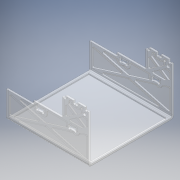
# Autodesk Inventor part: バッテリーボックス底板
Saved by Autodesk Inventor 2016 (Build 200138000, 138)
## iProperties
Created: 2019-03-23
Part Number: バッテリーボックス底板
Material: ポリカーボネート、クリア
Document SubType Name: Modeling
Designer: mozar
Density: 1.2 g/cm^3
Appearance: ポリカーボネート - クリア
Author: mozar
Autodesk Inventor part; units mm, degrees
note: some values were not read from the file. Chosen so that the rebuilt part matches the saved one: bend side of "曲げパーツ2".
(part 1 of 2)
ref_plane "YZ Plane" through (0, 0, 0) normal (1, 0, 0) x (0, 1, 0)
ref_plane "XZ Plane" through (0, 0, 0) normal (0, 1, 0) x (-1, 0, 0)
ref_plane "XY Plane" through (0, 0, 0) normal (0, 0, 1) x (1, 0, 0)
sketch "スケッチ1" plane through (0, 0, 0) normal (0, 0, 1) x (1, 0, 0)
  circle A0 centre (140, 30) radius 1.5
  circle A1 centre (140, -164.2) radius 1.5
  arc A2 (140.8182, -159.775) -> (142, -158.7917) centre (141, -158.7917) ccw
  line L0 (142, -158.7917) -> (142, -151.9032)
  arc A3 (142, -151.9032) -> (140.4377, -151.0763) centre (141, -151.9032) ccw
  line L1 (140.4377, -151.0763) -> (133.3836, -155.8731)
  arc A4 (133.3836, -155.8731) -> (133.3836, -157.5269) centre (133.9459, -156.7) ccw
  line L2 (133.3836, -157.5269) -> (137.0951, -160.0507)
  arc A5 (137.0951, -160.0507) -> (138.0834, -160.1286) centre (137.6574, -159.2238) ccw
  arc A6 (140.8182, -159.775) -> (138.0834, -160.1286) centre (140, -164.2) ccw
  arc A7 (136.2251, -169.2) -> (136.9114, -167.4727) centre (136.2251, -168.2) ccw
  arc A8 (136.7273, -167.2886) -> (136.9114, -167.4727) centre (140, -164.2) ccw
  arc A9 (136.7273, -167.2886) -> (135, -167.9749) centre (136, -167.9749) ccw
  line L3 (135, -167.9749) -> (135, -168.2)
  arc A10 (135, -168.2) -> (136, -169.2) centre (136, -168.2) ccw
  line L4 (136, -169.2) -> (136.2251, -169.2)
  arc A11 (136.9114, 33.2727) -> (136.2251, 35) centre (136.2251, 34) ccw
  line L5 (136.2251, 35) -> (136, 35)
  arc A12 (136, 35) -> (135, 34) centre (136, 34) ccw
  line L6 (135, 34) -> (135, 33.7749)
  arc A13 (135, 33.7749) -> (136.7273, 33.0886) centre (136, 33.7749) ccw
  arc A14 (136.9114, 33.2727) -> (136.7273, 33.0886) centre (140, 30) ccw
  arc A15 (140.4377, 16.8763) -> (142, 17.7032) centre (141, 17.7032) ccw
  line L7 (142, 17.7032) -> (142, 24.5917)
  arc A16 (142, 24.5917) -> (140.8182, 25.575) centre (141, 24.5917) ccw
  arc A17 (138.0834, 25.9286) -> (140.8182, 25.575) centre (140, 30) ccw
  arc A18 (138.0834, 25.9286) -> (137.0951, 25.8507) centre (137.6574, 25.0238) ccw
  line L8 (137.0951, 25.8507) -> (133.3836, 23.3269)
  arc A19 (133.3836, 23.3269) -> (133.3836, 21.6731) centre (133.9459, 22.5) ccw
  line L9 (133.3836, 21.6731) -> (140.4377, 16.8763)
  arc A20 (130.0623, 20.3037) -> (128.9377, 20.3037) centre (129.5, 19.4768) ccw
  line L10 (128.9377, 20.3037) -> (122.3542, 15.8269)
  arc A21 (122.3542, 15.8269) -> (122.9165, 14) centre (122.9165, 15) ccw
  line L11 (122.9165, 14) -> (136.0835, 14)
  arc A22 (136.0835, 14) -> (136.6458, 15.8269) centre (136.0835, 15) ccw
  line L12 (136.6458, 15.8269) -> (130.0623, 20.3037)
  arc A23 (121, 32) -> (120.7896, 30.237) centre (121.3519, 31.064) ccw
  line L13 (120.7896, 30.237) -> (128.9377, 24.6963)
  arc A24 (128.9377, 24.6963) -> (130.0623, 24.6963) centre (129.5, 25.5232) ccw
  line L14 (130.0623, 24.6963) -> (135.1564, 28.1603)
  arc A25 (135.1564, 28.1603) -> (135.577, 29.1713) centre (134.5941, 28.9872) ccw
  arc A26 (135.575, 30.8182) -> (135.577, 29.1713) centre (140, 30) ccw
  arc A27 (135.575, 30.8182) -> (134.5917, 32) centre (134.5917, 31) ccw
  line L15 (134.5917, 32) -> (134, 32)
  arc A28 (134, 32) -> (133.4, 31.8) centre (134, 31) ccw
  arc A29 (129.8, 31.1842) -> (133.4, 31.8) centre (131, 35) ccw
  arc A30 (129.8, 31.1842) -> (129.2, 31.1842) centre (129.5, 30.2303) ccw
  arc A31 (125.6, 31.8) -> (129.2, 31.1842) centre (128, 35) ccw
  arc A32 (125.6, 31.8) -> (125, 32) centre (125, 31) ccw
  line L16 (125, 32) -> (124, 32)
  line L17 (124, 32) -> (124, 34)
  arc A33 (124, 34) -> (123, 35) centre (123, 34) ccw
  line L18 (123, 35) -> (122, 35)
  arc A34 (122, 35) -> (121, 34) centre (122, 34) ccw
  line L19 (121, 34) -> (121, 32)
  arc A35 (117, 17.7032) -> (118.5623, 16.8763) centre (118, 17.7032) ccw
  line L20 (118.5623, 16.8763) -> (125.6164, 21.6731)
  arc A36 (125.6164, 21.6731) -> (125.6164, 23.3269) centre (125.0541, 22.5) ccw
  line L21 (125.6164, 23.3269) -> (118.5623, 28.1237)
  arc A37 (118.5623, 28.1237) -> (117, 27.2968) centre (118, 27.2968) ccw
  line L22 (117, 27.2968) -> (117, 17.7032)
  arc A38 (125, 4) -> (124.4, 3.8) centre (125, 3) ccw
  arc A39 (121.6491, 3.0154) -> (124.4, 3.8) centre (122, 7) ccw
  arc A40 (121.6491, 3.0154) -> (121.2641, 2.9741) centre (121.5614, 2.0193) ccw
  line L23 (121.2641, 2.9741) -> (101.9364, -3.0425)
  arc A41 (101.9364, -3.0425) -> (101.9774, -4.9639) centre (102.2336, -3.9973) ccw
  line L24 (101.9774, -4.9639) -> (140.7437, -15.2421)
  arc A42 (140.7437, -15.2421) -> (142, -14.2755) centre (141, -14.2755) ccw
  line L25 (142, -14.2755) -> (142, 8.0704)
  arc A43 (142, 8.0704) -> (140.7028, 9.0252) centre (141, 8.0704) ccw
  line L26 (140.7028, 9.0252) -> (133.5686, 6.8044)
  arc A44 (133.5686, 6.8044) -> (132.8927, 6.0797) centre (133.8659, 5.8496) ccw
  arc A45 (126.6, 3.8) -> (132.8927, 6.0797) centre (129, 7) ccw
  arc A46 (126.6, 3.8) -> (126, 4) centre (126, 3) ccw
  line L27 (126, 4) -> (125, 4)
  arc A47 (80.0808, 6.2) -> (79.101, 7) centre (79.101, 6) ccw
  line L28 (79.101, 7) -> (64.5268, 7)
  arc A48 (64.5268, 7) -> (64.2705, 5.0334) centre (64.5268, 6) ccw
  line L29 (64.2705, 5.0334) -> (92.8926, -2.5553)
  arc A49 (92.8926, -2.5553) -> (93.4461, -2.5435) centre (93.1489, -1.5887) ccw
  line L30 (93.4461, -2.5435) -> (117.4252, 4.9211)
  arc A50 (117.4252, 4.9211) -> (118.1024, 6.1007) centre (117.128, 5.8759) ccw
  arc A51 (118, 7) -> (118.1024, 6.1007) centre (122, 7) ccw
  line L31 (118, 7) -> (118, 10)
  arc A52 (118, 10) -> (117, 11) centre (117, 10) ccw
  line L32 (117, 11) -> (96, 11)
  arc A53 (96, 11) -> (95, 10) centre (96, 10) ccw
  line L33 (95, 10) -> (95, 7)
  arc A54 (88.6, 3.8) -> (95, 7) centre (91, 7) ccw
  arc A55 (88.6, 3.8) -> (88, 4) centre (88, 3) ccw
  line L34 (88, 4) -> (87, 4)
  arc A56 (87, 4) -> (86.4, 3.8) centre (87, 3) ccw
  arc A57 (80.0808, 6.2) -> (86.4, 3.8) centre (84, 7) ccw
  arc A58 (52.2563, 5.1151) -> (51, 4.1485) centre (52, 4.1485) ccw
  line L35 (51, 4.1485) -> (51, -14.398)
  arc A59 (51, -14.398) -> (52.2972, -15.3528) centre (52, -14.398) ccw
  line L36 (52.2972, -15.3528) -> (84.4723, -5.337)
  arc A60 (84.4723, -5.337) -> (84.4313, -3.4155) centre (84.1751, -4.3821) ccw
  line L37 (84.4313, -3.4155) -> (52.2563, 5.1151)
  arc A61 (127.9942, -17) -> (128.2505, -15.0334) centre (127.9942, -16) ccw
  line L38 (128.2505, -15.0334) -> (93.5161, -5.8242)
  arc A62 (93.5161, -5.8242) -> (92.9626, -5.836) centre (93.2598, -6.7908) ccw
  line L39 (92.9626, -5.836) -> (63.3788, -15.0452)
  arc A63 (63.3788, -15.0452) -> (63.676, -17) centre (63.676, -16) ccw
  line L40 (63.676, -17) -> (127.9942, -17)
  arc A64 (128.2505, -119.1666) -> (127.9942, -117.2) centre (127.9942, -118.2) ccw
  line L41 (127.9942, -117.2) -> (63.1515, -117.2)
  arc A65 (63.1515, -117.2) -> (62.8561, -119.1554) centre (63.1515, -118.2) ccw
  line L42 (62.8561, -119.1554) -> (92.7876, -128.4114)
  arc A66 (92.7876, -128.4114) -> (93.3393, -128.4227) centre (93.0831, -127.4561) ccw
  line L43 (93.3393, -128.4227) -> (128.2505, -119.1666)
  arc A67 (51, -138.3485) -> (52.2563, -139.3151) centre (52, -138.3485) ccw
  line L44 (52.2563, -139.3151) -> (84.2275, -130.8385)
  arc A68 (84.2275, -130.8385) -> (84.2666, -128.9165) centre (83.9712, -129.8719) ccw
  line L45 (84.2666, -128.9165) -> (52.2954, -119.0297)
  arc A69 (52.2954, -119.0297) -> (51, -119.9851) centre (52, -119.9851) ccw
  line L46 (51, -119.9851) -> (51, -138.3485)
  arc A70 (123, -169.2) -> (124, -168.2) centre (123, -168.2) ccw
  line L47 (124, -168.2) -> (124, -166.2)
  line L48 (124, -166.2) -> (125, -166.2)
  arc A71 (125, -166.2) -> (125.6, -166) centre (125, -165.2) ccw
  arc A72 (129.2, -165.3842) -> (125.6, -166) centre (128, -169.2) ccw
  arc A73 (129.2, -165.3842) -> (129.8, -165.3842) centre (129.5, -164.4303) ccw
  arc A74 (133.4, -166) -> (129.8, -165.3842) centre (131, -169.2) ccw
  arc A75 (133.4, -166) -> (134, -166.2) centre (134, -165.2) ccw
  line L49 (134, -166.2) -> (134.5917, -166.2)
  arc A76 (134.5917, -166.2) -> (135.575, -165.0182) centre (134.5917, -165.2) ccw
  arc A77 (135.577, -163.3713) -> (135.575, -165.0182) centre (140, -164.2) ccw
  arc A78 (135.577, -163.3713) -> (135.1564, -162.3603) centre (134.5941, -163.1872) ccw
  line L50 (135.1564, -162.3603) -> (130.0623, -158.8963)
  arc A79 (130.0623, -158.8963) -> (128.9377, -158.8963) centre (129.5, -159.7232) ccw
  line L51 (128.9377, -158.8963) -> (120.7896, -164.437)
  arc A80 (120.7896, -164.437) -> (121, -166.2) centre (121.3519, -165.264) ccw
  line L52 (121, -166.2) -> (121, -168.2)
  arc A81 (121, -168.2) -> (122, -169.2) centre (122, -168.2) ccw
  line L53 (122, -169.2) -> (123, -169.2)
  arc A82 (125.6164, -157.5269) -> (125.6164, -155.8731) centre (125.0541, -156.7) ccw
  line L54 (125.6164, -155.8731) -> (118.5623, -151.0763)
  arc A83 (118.5623, -151.0763) -> (117, -151.9032) centre (118, -151.9032) ccw
  line L55 (117, -151.9032) -> (117, -161.4968)
  arc A84 (117, -161.4968) -> (118.5623, -162.3237) centre (118, -161.4968) ccw
  line L56 (118.5623, -162.3237) -> (125.6164, -157.5269)
  arc A85 (122.9165, -148.2) -> (122.3542, -150.0269) centre (122.9165, -149.2) ccw
  line L57 (122.3542, -150.0269) -> (128.9377, -154.5037)
  arc A86 (128.9377, -154.5037) -> (130.0623, -154.5037) centre (129.5, -153.6768) ccw
  line L58 (130.0623, -154.5037) -> (136.6458, -150.0269)
  arc A87 (136.6458, -150.0269) -> (136.0835, -148.2) centre (136.0835, -149.2) ccw
  line L59 (136.0835, -148.2) -> (122.9165, -148.2)
  arc A88 (121.1595, -137.1852) -> (121.5639, -137.2238) centre (121.4549, -136.2298) ccw
  arc A89 (124.4, -138) -> (121.5639, -137.2238) centre (122, -141.2) ccw
  arc A90 (124.4, -138) -> (125, -138.2) centre (125, -137.2) ccw
  line L60 (125, -138.2) -> (126, -138.2)
  arc A91 (126, -138.2) -> (126.6, -138) centre (126, -137.2) ccw
  arc A92 (132.8964, -140.2954) -> (126.6, -138) centre (129, -141.2) ccw
  arc A93 (132.8964, -140.2954) -> (133.575, -141.0246) centre (133.8705, -140.0692) ccw
  line L61 (133.575, -141.0246) -> (140.7046, -143.2293)
  arc A94 (140.7046, -143.2293) -> (142, -142.2739) centre (141, -142.2739) ccw
  line L62 (142, -142.2739) -> (142, -119.9245)
  arc A95 (142, -119.9245) -> (140.7437, -118.9579) centre (141, -119.9245) ccw
  line L63 (140.7437, -118.9579) -> (101.8327, -129.2745)
  arc A96 (101.8327, -129.2745) -> (101.7935, -131.1964) centre (102.089, -130.2411) ccw
  line L64 (101.7935, -131.1964) -> (121.1595, -137.1852)
  arc A97 (117, -145.2) -> (118, -144.2) centre (117, -144.2) ccw
  line L65 (118, -144.2) -> (118, -141.2)
  arc A98 (118.094, -140.3377) -> (118, -141.2) centre (122, -141.2) ccw
  arc A99 (118.094, -140.3377) -> (117.413, -139.1668) centre (117.1176, -140.1221) ccw
  line L66 (117.413, -139.1668) -> (93.2725, -131.7015)
  arc A100 (93.2725, -131.7015) -> (92.7208, -131.6903) centre (92.9771, -132.6569) ccw
  line L67 (92.7208, -131.6903) -> (64.2705, -139.2334)
  arc A101 (64.2705, -139.2334) -> (64.5268, -141.2) centre (64.5268, -140.2) ccw
  line L68 (64.5268, -141.2) -> (79.101, -141.2)
  arc A102 (79.101, -141.2) -> (80.0808, -140.4) centre (79.101, -140.2) ccw
  arc A103 (86.4, -138) -> (80.0808, -140.4) centre (84, -141.2) ccw
  arc A104 (86.4, -138) -> (87, -138.2) centre (87, -137.2) ccw
  line L69 (87, -138.2) -> (88, -138.2)
  arc A105 (88, -138.2) -> (88.6, -138) centre (88, -137.2) ccw
  arc A106 (95, -141.2) -> (88.6, -138) centre (91, -141.2) ccw
  line L70 (95, -141.2) -> (95, -144.2)
  arc A107 (95, -144.2) -> (96, -145.2) centre (96, -144.2) ccw
  line L71 (96, -145.2) -> (117, -145.2)
  arc A108 (128, -144.2) -> (130, -144.2) centre (129, -144.2) ccw
  line L72 (130, -144.2) -> (130, -141.2)
  arc A109 (130, -141.2) -> (128, -141.2) centre (129, -141.2) ccw
  line L73 (128, -141.2) -> (123, -141.2)
  arc A110 (123, -141.2) -> (121, -141.2) centre (122, -141.2) ccw
  line L74 (121, -141.2) -> (121, -144.2)
  arc A111 (121, -144.2) -> (123, -144.2) centre (122, -144.2) ccw
  line L75 (123, -144.2) -> (128, -144.2)
  arc A112 (90, 7) -> (92, 7) centre (91, 7) ccw
  line L76 (92, 7) -> (92, 10)
  arc A113 (92, 10) -> (90, 10) centre (91, 10) ccw
  line L77 (90, 10) -> (85, 10)
  arc A114 (85, 10) -> (83, 10) centre (84, 10) ccw
  line L78 (83, 10) -> (83, 7)
  arc A115 (83, 7) -> (85, 7) centre (84, 7) ccw
  line L79 (85, 7) -> (90, 7)
  arc A116 (121, 7) -> (123, 7) centre (122, 7) ccw
  line L80 (123, 7) -> (128, 7)
  arc A117 (128, 7) -> (130, 7) centre (129, 7) ccw
  line L81 (130, 7) -> (130, 10)
  arc A118 (130, 10) -> (128, 10) centre (129, 10) ccw
  line L82 (128, 10) -> (123, 10)
  arc A119 (123, 10) -> (121, 10) centre (122, 10) ccw
  line L83 (121, 10) -> (121, 7)
  arc A120 (83, -144.2) -> (85, -144.2) centre (84, -144.2) ccw
  line L84 (85, -144.2) -> (90, -144.2)
  arc A121 (90, -144.2) -> (92, -144.2) centre (91, -144.2) ccw
  line L85 (92, -144.2) -> (92, -141.2)
  arc A122 (92, -141.2) -> (90, -141.2) centre (91, -141.2) ccw
  line L86 (90, -141.2) -> (85, -141.2)
  arc A123 (85, -141.2) -> (83, -141.2) centre (84, -141.2) ccw
  line L87 (83, -141.2) -> (83, -144.2)
  arc A124 (24.5071, -36.0492) -> (23.2695, -35.6053) centre (23.6339, -36.5366) ccw
  line L88 (23.2695, -35.6053) -> (2.9387, -43.5608)
  arc A125 (2.9387, -43.5608) -> (3.0119, -45.4487) centre (3.3031, -44.4921) ccw
  line L89 (3.0119, -45.4487) -> (22.9517, -51.5174)
  arc A126 (22.9517, -51.5174) -> (24.1943, -50.8686) centre (23.2428, -50.5607) ccw
  arc A127 (25.7746, -48.7762) -> (24.1943, -50.8686) centre (28, -52.1) ccw
  line L90 (25.7746, -48.7762) -> (26, -48.1)
  line L91 (26, -48.1) -> (32, -48.1)
  arc A128 (32, -48.1) -> (33, -47.1) centre (32, -47.1) ccw
  line L92 (33, -47.1) -> (33, -39.1)
  arc A129 (33, -39.1) -> (32, -38.1) centre (32, -39.1) ccw
  line L93 (32, -38.1) -> (26, -38.1)
  line L94 (26, -38.1) -> (25.8761, -37.7283)
  arc A130 (25.8761, -37.7283) -> (25.5419, -37.2556) centre (24.9274, -38.0445) ccw
  arc A131 (24.5071, -36.0492) -> (25.5419, -37.2556) centre (28, -34.1) ccw
  arc A132 (-24.4188, -35.8819) -> (-23.8147, -37.2841) centre (-23.5236, -36.3274) ccw
  line L95 (-23.8147, -37.2841) -> (-4.7062, -43.0997)
  arc A133 (-4.7062, -43.0997) -> (-4.0507, -43.0743) centre (-4.4151, -42.1431) ccw
  line L96 (-4.0507, -43.0743) -> (12.6705, -36.5312)
  arc A134 (12.6705, -36.5312) -> (12.3061, -34.6) centre (12.3061, -35.6) ccw
  line L97 (12.3061, -34.6) -> (-23.2303, -34.6)
  arc A135 (-23.2303, -34.6) -> (-24.1842, -35.3) centre (-23.2303, -35.6) ccw
  arc A136 (-24.4188, -35.8819) -> (-24.1842, -35.3) centre (-28, -34.1) ccw
  arc A137 (-3.9188, -46.4753) -> (-4.5743, -46.5007) centre (-4.2099, -47.4319) ccw
  line L98 (-4.5743, -46.5007) -> (-12.6705, -49.6688)
  arc A138 (-12.6705, -49.6688) -> (-12.3061, -51.6) centre (-12.3061, -50.6) ccw
  line L99 (-12.3061, -51.6) -> (6.1994, -51.6)
  arc A139 (6.1994, -51.6) -> (6.4906, -49.6433) centre (6.1994, -50.6) ccw
  line L100 (6.4906, -49.6433) -> (-3.9188, -46.4753)
  arc A140 (-24.5071, -50.1508) -> (-23.2695, -50.5947) centre (-23.6339, -49.6634) ccw
  line L101 (-23.2695, -50.5947) -> (-11.5637, -46.0142)
  arc A141 (-11.5637, -46.0142) -> (-11.6369, -44.1263) centre (-11.9281, -45.0829) ccw
  line L102 (-11.6369, -44.1263) -> (-28.7088, -38.9305)
  arc A142 (-28.7088, -38.9305) -> (-30, -39.8871) centre (-29, -39.8871) ccw
  line L103 (-30, -39.8871) -> (-30, -40.1)
  line L104 (-30, -40.1) -> (-32, -40.1)
  arc A143 (-32, -40.1) -> (-33, -41.1) centre (-32, -41.1) ccw
  line L105 (-33, -41.1) -> (-33, -47.1)
  arc A144 (-33, -47.1) -> (-32, -48.1) centre (-32, -47.1) ccw
  line L106 (-32, -48.1) -> (-26, -48.1)
  line L107 (-26, -48.1) -> (-25.8761, -48.4717)
  arc A145 (-25.8761, -48.4717) -> (-25.5419, -48.9444) centre (-24.9274, -48.1555) ccw
  arc A146 (-24.5071, -50.1508) -> (-25.5419, -48.9444) centre (-28, -52.1) ccw
  arc A147 (-44.8158, -35.3) -> (-45.7697, -34.6) centre (-45.7697, -35.6) ccw
  line L108 (-45.7697, -34.6) -> (-49, -34.6)
  line L109 (-49, -34.6) -> (-49, -50.6)
  arc A148 (-49, -50.6) -> (-48, -51.6) centre (-48, -50.6) ccw
  line L110 (-48, -51.6) -> (-45.7697, -51.6)
  arc A149 (-45.7697, -51.6) -> (-44.8158, -50.9) centre (-45.7697, -50.6) ccw
  arc A150 (-43.4581, -48.9444) -> (-44.8158, -50.9) centre (-41, -52.1) ccw
  arc A151 (-43.4581, -48.9444) -> (-43.1239, -48.4717) centre (-44.0726, -48.1555) ccw
  line L111 (-43.1239, -48.4717) -> (-43, -48.1)
  line L112 (-43, -48.1) -> (-37, -48.1)
  arc A152 (-37, -48.1) -> (-36, -47.1) centre (-37, -47.1) ccw
  line L113 (-36, -47.1) -> (-36, -41.1)
  arc A153 (-36, -41.1) -> (-37, -40.1) centre (-37, -41.1) ccw
  line L114 (-37, -40.1) -> (-39, -40.1)
  line L115 (-39, -40.1) -> (-39, -38.999)
  arc A154 (-39, -38.999) -> (-40.2, -38.0192) centre (-40, -38.999) ccw
  arc A155 (-44.8158, -35.3) -> (-40.2, -38.0192) centre (-41, -34.1) ccw
  arc A156 (-33.9671, -24.899) -> (-35.1671, -23.9192) centre (-34.9671, -24.899) ccw
  arc A157 (-38.3671, -23.2) -> (-35.1671, -23.9192) centre (-35.9671, -20) ccw
  arc A158 (-38.3671, -23.2) -> (-38.9671, -23) centre (-38.9671, -24) ccw
  line L116 (-38.9671, -23) -> (-48, -23)
  arc A159 (-48, -23) -> (-49, -24) centre (-48, -24) ccw
  line L117 (-49, -24) -> (-49, -29.6)
  arc A160 (-49, -29.6) -> (-48, -30.6) centre (-48, -29.6) ccw
  line L118 (-48, -30.6) -> (-45.7697, -30.6)
  arc A161 (-45.7697, -30.6) -> (-44.8158, -29.9) centre (-45.7697, -29.6) ccw
  arc A162 (-43.4581, -27.9444) -> (-44.8158, -29.9) centre (-41, -31.1) ccw
  arc A163 (-43.4581, -27.9444) -> (-43.1239, -27.4717) centre (-44.0726, -27.1555) ccw
  line L119 (-43.1239, -27.4717) -> (-43, -27.1)
  line L120 (-43, -27.1) -> (-34.962, -27.1)
  arc A164 (-34.962, -27.1) -> (-33.9671, -26) centre (-34.962, -26.1) ccw
  line L121 (-33.9671, -26) -> (-33.9671, -24.899)
  arc A165 (14.3908, -24.607) -> (15.2527, -25.1) centre (15.2527, -24.1) ccw
  line L122 (15.2527, -25.1) -> (44.4281, -25.1)
  arc A166 (44.4281, -25.1) -> (45.29, -24.607) centre (44.4281, -24.1) ccw
  line L123 (45.29, -24.607) -> (47.8619, -20.2347)
  line L124 (48, -19.7277) -> (48, 10)
  line L125 (48, 10) -> (79, 10)
  arc A167 (79, 10) -> (80, 11) centre (79, 11) ccw
  line L126 (80, 11) -> (80, 14)
  line L127 (80, 14) -> (113, 14)
  arc A168 (113, 14) -> (114, 15) centre (113, 15) ccw
  line L128 (114, 15) -> (114, 35)
  line L129 (114, 35) -> (116, 35)
  arc A169 (116, 35) -> (118, 35) centre (117, 35) ccw
  line L130 (118, 35) -> (118, 38)
  line L131 (118, 38) -> (127, 38)
  line L132 (127, 38) -> (127, 35)
  arc A170 (127, 35) -> (129, 35) centre (128, 35) ccw
  line L133 (129, 35) -> (130, 35)
  arc A171 (130, 35) -> (132, 35) centre (131, 35) ccw
  line L134 (132, 35) -> (132, 38)
  line L135 (132, 38) -> (141, 38)
  line L136 (141, 38) -> (141, 35)
  arc A172 (141, 35) -> (143, 35) centre (142, 35) ccw
  line L137 (143, 35) -> (145, 35)
  line L138 (145, 35) -> (145, -169.2)
  line L139 (145, -169.2) -> (143, -169.2)
  arc A173 (143, -169.2) -> (141, -169.2) centre (142, -169.2) ccw
  line L140 (141, -169.2) -> (141, -172.2)
  line L141 (141, -172.2) -> (132, -172.2)
  line L142 (132, -172.2) -> (132, -169.2)
  arc A174 (132, -169.2) -> (130, -169.2) centre (131, -169.2) ccw
  line L143 (130, -169.2) -> (129, -169.2)
  arc A175 (129, -169.2) -> (127, -169.2) centre (128, -169.2) ccw
  line L144 (127, -169.2) -> (127, -172.2)
  line L145 (127, -172.2) -> (118, -172.2)
  line L146 (118, -172.2) -> (118, -169.2)
  arc A176 (118, -169.2) -> (116, -169.2) centre (117, -169.2) ccw
  line L147 (116, -169.2) -> (114, -169.2)
  line L148 (114, -169.2) -> (114, -149.2)
  arc A177 (114, -149.2) -> (113, -148.2) centre (113, -149.2) ccw
  line L149 (113, -148.2) -> (80, -148.2)
  line L150 (80, -148.2) -> (80, -145.2)
  arc A178 (80, -145.2) -> (79, -144.2) centre (79, -145.2) ccw
  line L151 (79, -144.2) -> (48, -144.2)
  line L152 (48, -144.2) -> (48, -114.4723)
  line L153 (47.8619, -113.9653) -> (45.29, -109.593)
  arc A179 (45.29, -109.593) -> (44.4281, -109.1) centre (44.4281, -110.1) ccw
  line L154 (44.4281, -109.1) -> (15.2527, -109.1)
  arc A180 (15.2527, -109.1) -> (14.3908, -109.593) centre (15.2527, -110.1) ccw
  line L155 (14.3908, -109.593) -> (11.8189, -113.9653)
  arc A181 (11.8189, -113.9653) -> (11.6808, -114.4723) centre (12.6808, -114.4723) ccw
  line L156 (11.6808, -114.4723) -> (11.6808, -117.2)
  line L157 (11.6808, -117.2) -> (11.399, -117.2)
  arc A182 (11.399, -117.2) -> (10.4192, -118) centre (11.399, -118.2) ccw
  arc A183 (4.1, -120.4) -> (10.4192, -118) centre (6.5, -117.2) ccw
  arc A184 (4.1, -120.4) -> (3.5, -120.2) centre (3.5, -121.2) ccw
  line L158 (3.5, -120.2) -> (-3.5, -120.2)
  arc A185 (-3.5, -120.2) -> (-4.1, -120.4) centre (-3.5, -121.2) ccw
  arc A186 (-10.4192, -118) -> (-4.1, -120.4) centre (-6.5, -117.2) ccw
  arc A187 (-10.4192, -118) -> (-11.399, -117.2) centre (-11.399, -118.2) ccw
  line L159 (-11.399, -117.2) -> (-11.6808, -117.2)
  line L160 (-11.6808, -117.2) -> (-11.6808, -115.2)
  arc A188 (-11.6808, -115.2) -> (-12.6808, -114.2) centre (-12.6808, -115.2) ccw
  line L161 (-12.6808, -114.2) -> (-16.7863, -114.2)
  arc A189 (-16.7863, -114.2) -> (-17.7863, -115.2) centre (-16.7863, -115.2) ccw
  line L162 (-17.7863, -115.2) -> (-17.7863, -117.2)
  line L163 (-17.7863, -117.2) -> (-18.0681, -117.2)
  arc A190 (-18.0681, -117.2) -> (-19.0479, -118) centre (-18.0681, -118.2) ccw
  arc A191 (-25.3671, -120.4) -> (-19.0479, -118) centre (-22.9671, -117.2) ccw
  arc A192 (-25.3671, -120.4) -> (-25.9671, -120.2) centre (-25.9671, -121.2) ccw
  line L164 (-25.9671, -120.2) -> (-32.9671, -120.2)
  arc A193 (-32.9671, -120.2) -> (-33.5671, -120.4) centre (-32.9671, -121.2) ccw
  arc A194 (-39.8862, -118) -> (-33.5671, -120.4) centre (-35.9671, -117.2) ccw
  arc A195 (-39.8862, -118) -> (-40.866, -117.2) centre (-40.866, -118.2) ccw
  line L165 (-40.866, -117.2) -> (-41.1478, -117.2)
  line L166 (-41.1478, -117.2) -> (-41.1478, -115.2)
  arc A196 (-41.1478, -115.2) -> (-42.1478, -114.2) centre (-42.1478, -115.2) ccw
  line L167 (-42.1478, -114.2) -> (-52, -114.2)
  line L168 (-52, -114.2) -> (-52, -20)
  line L169 (-52, -20) -> (-42.1478, -20)
  arc A197 (-42.1478, -20) -> (-41.1478, -19) centre (-42.1478, -19) ccw
  line L170 (-41.1478, -19) -> (-41.1478, -17)
  line L171 (-41.1478, -17) -> (-40.866, -17)
  arc A198 (-40.866, -17) -> (-39.8862, -16.2) centre (-40.866, -16) ccw
  arc A199 (-33.5671, -13.8) -> (-39.8862, -16.2) centre (-35.9671, -17) ccw
  arc A200 (-33.5671, -13.8) -> (-32.9671, -14) centre (-32.9671, -13) ccw
  line L172 (-32.9671, -14) -> (-25.9671, -14)
  arc A201 (-25.9671, -14) -> (-25.3671, -13.8) centre (-25.9671, -13) ccw
  arc A202 (-19.0479, -16.2) -> (-25.3671, -13.8) centre (-22.9671, -17) ccw
  arc A203 (-19.0479, -16.2) -> (-18.0681, -17) centre (-18.0681, -16) ccw
  line L173 (-18.0681, -17) -> (-17.7863, -17)
  line L174 (-17.7863, -17) -> (-17.7863, -19)
  arc A204 (-17.7863, -19) -> (-16.7863, -20) centre (-16.7863, -19) ccw
  line L175 (-16.7863, -20) -> (-12.6808, -20)
  arc A205 (-12.6808, -20) -> (-11.6808, -19) centre (-12.6808, -19) ccw
  line L176 (-11.6808, -19) -> (-11.6808, -17)
  line L177 (-11.6808, -17) -> (-11.399, -17)
  arc A206 (-11.399, -17) -> (-10.4192, -16.2) centre (-11.399, -16) ccw
  arc A207 (-4.1, -13.8) -> (-10.4192, -16.2) centre (-6.5, -17) ccw
  arc A208 (-4.1, -13.8) -> (-3.5, -14) centre (-3.5, -13) ccw
  line L178 (-3.5, -14) -> (3.5, -14)
  arc A209 (3.5, -14) -> (4.1, -13.8) centre (3.5, -13) ccw
  arc A210 (10.4192, -16.2) -> (4.1, -13.8) centre (6.5, -17) ccw
  arc A211 (10.4192, -16.2) -> (11.399, -17) centre (11.399, -16) ccw
  line L179 (11.399, -17) -> (11.6808, -17)
  line L180 (11.6808, -17) -> (11.6808, -19.7277)
  arc A212 (11.6808, -19.7277) -> (11.8189, -20.2347) centre (12.6808, -19.7277) ccw
  line L181 (11.8189, -20.2347) -> (14.3908, -24.607)
  arc A213 (23.2303, -30.6) -> (24.1842, -29.9) centre (23.2303, -29.6) ccw
  arc A214 (24.3339, -29.5) -> (24.1842, -29.9) centre (28, -31.1) ccw
  arc A215 (24.3339, -29.5) -> (23.4174, -28.1) centre (23.4174, -29.1) ccw
  line L182 (23.4174, -28.1) -> (12.965, -28.1)
  line L183 (12.965, -28.1) -> (10.2873, -23.5479)
  arc A216 (10.2873, -23.5479) -> (8.8403, -23.2439) centre (9.4253, -24.0549) ccw
  arc A217 (5.7, -23.9192) -> (8.8403, -23.2439) centre (6.5, -20) ccw
  arc A218 (5.7, -23.9192) -> (4.5, -24.899) centre (5.5, -24.899) ccw
  line L184 (4.5, -24.899) -> (4.5, -26)
  line L185 (4.5, -26) -> (-4.5, -26)
  line L186 (-4.5, -26) -> (-4.5, -24.899)
  arc A219 (-4.5, -24.899) -> (-5.7, -23.9192) centre (-5.5, -24.899) ccw
  arc A220 (-8.9, -23.2) -> (-5.7, -23.9192) centre (-6.5, -20) ccw
  arc A221 (-8.9, -23.2) -> (-9.5, -23) centre (-9.5, -24) ccw
  line L187 (-9.5, -23) -> (-19.9671, -23)
  arc A222 (-19.9671, -23) -> (-20.5671, -23.2) centre (-19.9671, -24) ccw
  arc A223 (-23.7671, -23.9192) -> (-20.5671, -23.2) centre (-22.9671, -20) ccw
  arc A224 (-23.7671, -23.9192) -> (-24.9671, -24.899) centre (-23.9671, -24.899) ccw
  line L188 (-24.9671, -24.899) -> (-24.9671, -26)
  line L189 (-24.9671, -26) -> (-24.9792, -26)
  arc A225 (-24.9792, -26) -> (-25.9279, -27.3162) centre (-24.9792, -27) ccw
  line L190 (-25.9279, -27.3162) -> (-25.8761, -27.4717)
  arc A226 (-25.8761, -27.4717) -> (-25.5419, -27.9444) centre (-24.9274, -27.1555) ccw
  arc A227 (-24.1842, -29.9) -> (-25.5419, -27.9444) centre (-28, -31.1) ccw
  arc A228 (-24.1842, -29.9) -> (-23.2303, -30.6) centre (-23.2303, -29.6) ccw
  line L191 (-23.2303, -30.6) -> (23.2303, -30.6)
  circle A229 centre (34.5, -29.6) radius 1.5
  line L192 (34.5, -31.1) -> (29, -31.1)
  arc A230 (29, -31.1) -> (27, -31.1) centre (28, -31.1) ccw
  line L193 (27, -31.1) -> (27, -32.5348)
  line L194 (27, -32.5348) -> (27.5466, -33.9316)
  line L195 (27.5466, -33.9316) -> (27.001, -34.1451)
  arc A231 (27.001, -34.1451) -> (29, -34.1) centre (28, -34.1) ccw
  line L196 (29, -34.1) -> (40, -34.1)
  arc A232 (40, -34.1) -> (42, -34.1) centre (41, -34.1) ccw
  line L197 (42, -34.1) -> (42, -31.1)
  arc A233 (42, -31.1) -> (40, -31.1) centre (41, -31.1) ccw
  line L198 (40, -31.1) -> (34.5, -31.1)
  line L199 (-42, -52.1) -> (-42, -55.1)
  arc A234 (-42, -55.1) -> (-40, -55.1) centre (-41, -55.1) ccw
  line L200 (-40, -55.1) -> (-34.5, -55.1)
  circle A235 centre (-34.5, -56.6) radius 1.5
  line L201 (-34.5, -55.1) -> (-29, -55.1)
  arc A236 (-29, -55.1) -> (-27, -55.1) centre (-28, -55.1) ccw
  line L202 (-27, -55.1) -> (-27, -52.1)
  arc A237 (-27, -52.1) -> (-29, -52.1) centre (-28, -52.1) ccw
  line L203 (-29, -52.1) -> (-40, -52.1)
  arc A238 (-40, -52.1) -> (-42, -52.1) centre (-41, -52.1) ccw
  arc A239 (27, -55.1) -> (29, -55.1) centre (28, -55.1) ccw
  line L204 (29, -55.1) -> (34.5, -55.1)
  circle A240 centre (34.5, -56.6) radius 1.5
  line L205 (34.5, -55.1) -> (40, -55.1)
  arc A241 (40, -55.1) -> (42, -55.1) centre (41, -55.1) ccw
  line L206 (42, -55.1) -> (42, -52.1)
  arc A242 (42, -52.1) -> (40, -52.1) centre (41, -52.1) ccw
  line L207 (40, -52.1) -> (29, -52.1)
  arc A243 (29, -52.1) -> (27, -52.1) centre (28, -52.1) ccw
  line L208 (27, -52.1) -> (27, -55.1)
  line L209 (48, -51.6) -> (48, -55.6)
  line L210 (46.1514, -55.6) -> (45.7697, -55.6)
  arc A244 (45.7697, -55.6) -> (44.8158, -56.3) centre (45.7697, -56.6) ccw
  arc A245 (40.2, -59.0192) -> (44.8158, -56.3) centre (41, -55.1) ccw
  arc A246 (40.2, -59.0192) -> (39, -59.999) centre (40, -59.999) ccw
  line L211 (39, -59.999) -> (39, -61.1)
  line L212 (39, -61.1) -> (30, -61.1)
  line L213 (30, -61.1) -> (30, -59.999)
  arc A247 (30, -59.999) -> (28.8, -59.0192) centre (29, -59.999) ccw
  arc A248 (24.1842, -56.3) -> (28.8, -59.0192) centre (28, -55.1) ccw
  arc A249 (24.1842, -56.3) -> (23.2303, -55.6) centre (23.2303, -56.6) ccw
  line L214 (23.2303, -55.6) -> (-23.2303, -55.6)
  arc A250 (-23.2303, -55.6) -> (-24.1842, -56.3) centre (-23.2303, -56.6) ccw
  arc A251 (-28.8, -59.0192) -> (-24.1842, -56.3) centre (-28, -55.1) ccw
  arc A252 (-28.8, -59.0192) -> (-30, -59.999) centre (-29, -59.999) ccw
  line L215 (-30, -59.999) -> (-30, -61.1)
  line L216 (-30, -61.1) -> (-39, -61.1)
  line L217 (-39, -61.1) -> (-39, -59.999)
  arc A253 (-39, -59.999) -> (-40.2, -59.0192) centre (-40, -59.999) ccw
  arc A254 (-44.8158, -56.3) -> (-40.2, -59.0192) centre (-41, -55.1) ccw
  arc A255 (-44.8158, -56.3) -> (-45.7697, -55.6) centre (-45.7697, -56.6) ccw
  line L218 (-45.7697, -55.6) -> (-48, -55.6)
  arc A256 (-48, -55.6) -> (-49, -56.6) centre (-48, -56.6) ccw
  line L219 (-49, -56.6) -> (-49, -110.2)
  arc A257 (-49, -110.2) -> (-48, -111.2) centre (-48, -110.2) ccw
  line L220 (-48, -111.2) -> (-38.9671, -111.2)
  arc A258 (-38.9671, -111.2) -> (-38.3671, -111) centre (-38.9671, -110.2) ccw
  arc A259 (-35.1671, -110.2808) -> (-38.3671, -111) centre (-35.9671, -114.2) ccw
  arc A260 (-35.1671, -110.2808) -> (-33.9671, -109.301) centre (-34.9671, -109.301) ccw
  line L221 (-33.9671, -109.301) -> (-33.9671, -108.2)
  line L222 (-33.9671, -108.2) -> (-24.9671, -108.2)
  line L223 (-24.9671, -108.2) -> (-24.9671, -109.301)
  arc A261 (-24.9671, -109.301) -> (-23.7671, -110.2808) centre (-23.9671, -109.301) ccw
  arc A262 (-20.5671, -111) -> (-23.7671, -110.2808) centre (-22.9671, -114.2) ccw
  arc A263 (-20.5671, -111) -> (-19.9671, -111.2) centre (-19.9671, -110.2) ccw
  line L224 (-19.9671, -111.2) -> (-9.5205, -111.2)
  arc A264 (-9.5205, -111.2) -> (-8.918, -110.9981) centre (-9.5205, -110.2) ccw
  arc A265 (-5.7082, -110.2716) -> (-8.918, -110.9981) centre (-6.5082, -114.1907) ccw
  arc A266 (-5.7082, -110.2716) -> (-4.5082, -109.2918) centre (-5.5082, -109.2918) ccw
  line L225 (-4.5082, -109.2918) -> (-4.5082, -108.1907)
  line L226 (-4.5082, -108.1907) -> (4.4918, -108.1907)
  line L227 (4.4918, -108.1907) -> (4.4918, -109.2918)
  arc A267 (4.4918, -109.2918) -> (5.6918, -110.2716) centre (5.4918, -109.2918) ccw
  arc A268 (8.8397, -110.9523) -> (5.6918, -110.2716) centre (6.4918, -114.1907) ccw
  arc A269 (8.8397, -110.9523) -> (10.2886, -110.6497) centre (9.4267, -110.1427) ccw
  line L228 (10.2886, -110.6497) -> (12.965, -106.1)
  line L229 (12.965, -106.1) -> (46.7158, -106.1)
  line L230 (48.4805, -109.1) -> (49.4259, -110.707)
  arc A270 (49.4259, -110.707) -> (50.2878, -111.2) centre (50.2878, -110.2) ccw
  line L231 (50.2878, -111.2) -> (141, -111.2)
  arc A271 (141, -111.2) -> (142, -110.2) centre (141, -110.2) ccw
  line L232 (142, -110.2) -> (142, -24)
  arc A272 (142, -24) -> (141, -23) centre (141, -24) ccw
  line L233 (141, -23) -> (50.2878, -23)
  arc A273 (50.2878, -23) -> (49.4259, -23.493) centre (50.2878, -24) ccw
  line L234 (49.4259, -23.493) -> (48.4805, -25.1)
  line L235 (46.7158, -28.1) -> (45.5826, -28.1)
  arc A274 (45.5826, -28.1) -> (44.6661, -29.5) centre (45.5826, -29.1) ccw
  arc A275 (44.8158, -29.9) -> (44.6661, -29.5) centre (41, -31.1) ccw
  arc A276 (44.8158, -29.9) -> (45.7697, -30.6) centre (45.7697, -29.6) ccw
  line L236 (48, -30.6) -> (48, -34.6)
  arc A277 (45.7697, -34.6) -> (44.8158, -35.3) centre (45.7697, -35.6) ccw
  arc A278 (43.4581, -37.2556) -> (44.8158, -35.3) centre (41, -34.1) ccw
  arc A279 (43.4581, -37.2556) -> (43.1239, -37.7283) centre (44.0726, -38.0445) ccw
  line L237 (43.1239, -37.7283) -> (43, -38.1)
  line L238 (43, -38.1) -> (37, -38.1)
  arc A280 (37, -38.1) -> (36, -39.1) centre (37, -39.1) ccw
  line L239 (36, -39.1) -> (36, -47.1)
  arc A281 (36, -47.1) -> (37, -48.1) centre (37, -47.1) ccw
  line L240 (37, -48.1) -> (43, -48.1)
  line L241 (43, -48.1) -> (43.1239, -48.4717)
  arc A282 (43.1239, -48.4717) -> (43.4581, -48.9444) centre (44.0726, -48.1555) ccw
  arc A283 (44.8158, -50.9) -> (43.4581, -48.9444) centre (41, -52.1) ccw
  arc A284 (44.8158, -50.9) -> (45.7697, -51.6) centre (45.7697, -50.6) ccw
  line L242 (-7.5, -17) -> (-7.5, -20)
  arc A285 (-7.5, -20) -> (-5.5, -20) centre (-6.5, -20) ccw
  line L243 (-5.5, -20) -> (0, -20)
  line L244 (0, -20) -> (5.5, -20)
  arc A286 (5.5, -20) -> (7.5, -20) centre (6.5, -20) ccw
  line L245 (7.5, -20) -> (7.5, -17)
  arc A287 (7.5, -17) -> (5.5, -17) centre (6.5, -17) ccw
  line L246 (5.5, -17) -> (-5.5, -17)
  arc A288 (-5.5, -17) -> (-7.5, -17) centre (-6.5, -17) ccw
  circle A289 centre (0, -21.5) radius 1.5
  arc A290 (7.4918, -114.1907) -> (5.4918, -114.1907) centre (6.4918, -114.1907) ccw
  line L247 (5.4918, -114.1907) -> (-0.0082, -114.1907)
  arc A291 (-0.0082, -114.1907) -> (0.1582, -111.2) centre (-0.0082, -112.6907) ccw
  line L248 (0.1582, -111.2) -> (-0.1745, -111.2)
  arc A292 (-0.1745, -111.2) -> (-0.0082, -114.1907) centre (-0.0082, -112.6907) ccw
  line L249 (-0.0082, -114.1907) -> (-5.5082, -114.1907)
  arc A293 (-5.5082, -114.1907) -> (-7.5082, -114.1907) centre (-6.5082, -114.1907) ccw
  line L250 (-7.5082, -114.1907) -> (-7.5082, -117.1907)
  arc A294 (-7.5082, -117.1907) -> (-5.5082, -117.1907) centre (-6.5082, -117.1907) ccw
  line L251 (-5.5082, -117.1907) -> (5.4918, -117.1907)
  arc A295 (5.4918, -117.1907) -> (7.4918, -117.1907) centre (6.4918, -117.1907) ccw
  line L252 (7.4918, -117.1907) -> (7.4918, -114.1907)
  line L253 (-21.9671, -20) -> (-21.9671, -17)
  arc A296 (-21.9671, -17) -> (-23.9671, -17) centre (-22.9671, -17) ccw
  line L254 (-23.9671, -17) -> (-34.9671, -17)
  arc A297 (-34.9671, -17) -> (-36.9671, -17) centre (-35.9671, -17) ccw
  line L255 (-36.9671, -17) -> (-36.9671, -20)
  arc A298 (-36.9671, -20) -> (-34.9671, -20) centre (-35.9671, -20) ccw
  line L256 (-34.9671, -20) -> (-29.4671, -20)
  line L257 (-29.4671, -20) -> (-23.9671, -20)
  arc A299 (-23.9671, -20) -> (-21.9671, -20) centre (-22.9671, -20) ccw
  circle A300 centre (-29.4671, -21.5) radius 1.5
  line L258 (-23.9671, -114.2) -> (-29.4671, -114.2)
  circle A301 centre (-29.4671, -112.7) radius 1.5
  line L259 (-29.4671, -114.2) -> (-34.9671, -114.2)
  arc A302 (-34.9671, -114.2) -> (-36.9671, -114.2) centre (-35.9671, -114.2) ccw
  line L260 (-36.9671, -114.2) -> (-36.9671, -117.2)
  arc A303 (-36.9671, -117.2) -> (-34.9671, -117.2) centre (-35.9671, -117.2) ccw
  line L261 (-34.9671, -117.2) -> (-23.9671, -117.2)
  arc A304 (-23.9671, -117.2) -> (-21.9671, -117.2) centre (-22.9671, -117.2) ccw
  line L262 (-21.9671, -117.2) -> (-21.9671, -114.2)
  arc A305 (-21.9671, -114.2) -> (-23.9671, -114.2) centre (-22.9671, -114.2) ccw
  line L263 (-29, -31.1) -> (-40, -31.1)
  arc A306 (-40, -31.1) -> (-42, -31.1) centre (-41, -31.1) ccw
  line L264 (-42, -31.1) -> (-42, -34.1)
  arc A307 (-42, -34.1) -> (-40, -34.1) centre (-41, -34.1) ccw
  line L265 (-40, -34.1) -> (-34.5, -34.1)
  circle A308 centre (-34.5, -35.6) radius 1.5
  line L266 (-34.5, -34.1) -> (-29, -34.1)
  arc A309 (-29, -34.1) -> (-27, -34.1) centre (-28, -34.1) ccw
  line L267 (-27, -34.1) -> (-27, -31.1)
  arc A310 (-27, -31.1) -> (-29, -31.1) centre (-28, -31.1) ccw
  line L268 (48, -19.7277) -> (48, -114.4723)
  point P0 (0, 0)
  point P1 (0, 0)
  constraints: 604 point on circle, 538 end point, 304 centre point, 118 horizontal, 90 vertical, 7 vertical alignment, 3 point on line, 1 collinear, 1258 other
extrude "押し出し1" add sketch "スケッチ1" along normal blind 2 contours L124 L125 A167 L126 L127 A168 L128 L129 A169 L130 L131 L132 A170 L133 A171 L134 L135 L136 A172 L137 L138 L139 A173 L140 L141 L142 A174 L143 A175 L144 L145 L146 A176 L147 L148 A177 L149 L150 A178 L151 L152 L268 L209 L236